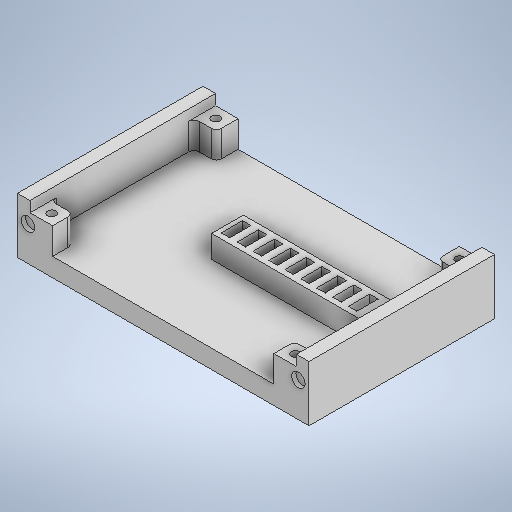
# Autodesk Inventor part: DisplayModuleHousing
Saved by Autodesk Inventor 2025.1 (Build 291241020, 241B)
## iProperties
Created: 2024-09-25
Part Number: DisplayModuleHousing
Material: Generic
Document SubType Name: Modeling
Designer: Si Teng Wu
Density: 1 g/cm^3
Appearance: Default
Author: Si Teng Wu
Autodesk Inventor part; units mm, degrees
ref_plane "YZ Plane" through (0, 0, 0) normal (1, 0, 0) x (0, 1, 0)
ref_plane "XZ Plane" through (0, 0, 0) normal (0, 1, 0) x (-1, 0, 0)
ref_plane "XY Plane" through (0, 0, 0) normal (0, 0, 1) x (1, 0, 0)
sketch "Sketch1" plane through (0, 0, 0) normal (0, 1, 0) x (-1, 0, 0)
  line L0 (55, 35) -> (-55, 35)
  line L1 (-55, 35) -> (-55, -35)
  line L2 (-55, -35) -> (55, -35)
  line L3 (55, -35) -> (55, 35)
  point P0 (0, 0)
  point P1 (-55, 0)
  point P2 (55, 0)
  dimension "d0" = 70
  dimension "d66" = 35
  dimension "d67" = 55
  dimension "d68" = 55
  constraints: 8 end point, 2 midpoint, 2 parallel, 1 horizontal, 1 perpendicular
  measures "d0" distance between parallel lines of L2 L0
  measures "d66" distance from line of L2 point (0, 0)
  measures "d67" distance of point (-55, 0) point (0, 0)
  measures "d68" distance of point (55, 0) point (0, 0)
extrude "Extrusion1" add sketch "Sketch1" along normal blind 21
sketch "Sketch2" plane through (0, 21, 0) normal (0, 1, 0) x (1, 0, 0)
  line L0 (-55, -35) -> (55, -35) projected
  line L1 (55, 35) -> (-55, 35) projected
  line L2 (50.25, -35) -> (-50.25, -35)
  line L3 (-50.25, -35) -> (-50.25, 35)
  line L4 (-50.25, 35) -> (50.25, 35)
  line L5 (50.25, 35) -> (50.25, -35)
  line L6 (-55, 35) -> (-55, -35) projected
  line L7 (55, -35) -> (55, 35) projected
  point P0 (0, 0)
  point P1 (-50.25, -35)
  dimension "d4" = 100.5
  dimension "d6" = 70
  dimension "d122" = 50.25
  constraints: 8 end point, 2 parallel, 2 point on line, 1 horizontal, 1 perpendicular
  measures "d4" distance between parallel lines of L3 L5
  measures "d6" distance between parallel lines of L1 L0
  measures "d122" distance from line of L3 point (0, 0)
extrude "Extrusion2" cut sketch "Sketch2" against normal blind 14 contours L3 L1 L5 L0
sketch "Sketch11" plane through (0, 7, 0) normal (0, 1, 0) x (1, 0, 0)
  line L0 (50.25, 35) -> (41.75, 35)
  line L1 (41.75, 35) -> (41.75, 26.8)
  line L2 (41.75, 26.8) -> (50.25, 26.8)
  line L3 (50.25, 26.8) -> (50.25, 35)
  circle A0 centre (46, 30.9) radius 1.6
  line L4 (50.25, 35) -> (50.25, -35) projected
  line L5 (50.25, -35) -> (41.75, -35)
  line L6 (41.75, -35) -> (41.75, -27.2)
  line L7 (41.75, -27.2) -> (50.25, -27.2)
  line L8 (50.25, -27.2) -> (50.25, -35)
  circle A1 centre (46, -31.1) radius 1.6
  line L9 (-41.75, 35) -> (-50.25, 35)
  line L10 (-50.25, 35) -> (-50.25, 26.8)
  line L11 (-50.25, 26.8) -> (-41.75, 26.8)
  line L12 (-41.75, 26.8) -> (-41.75, 35)
  circle A2 centre (-46, 30.8) radius 1.6
  line L13 (-50.25, 35) -> (50.25, 35) projected
  line L14 (-50.25, -35) -> (-50.25, 35) projected
  line L15 (-41.75, -35) -> (-50.25, -35)
  line L16 (-50.25, -35) -> (-50.25, -27.2)
  line L17 (-50.25, -27.2) -> (-41.75, -27.2)
  line L18 (-41.75, -27.2) -> (-41.75, -35)
  circle A3 centre (-46, -31.1) radius 1.6
  line L19 (50.25, -35) -> (-50.25, -35) projected
  point P0 (0, 0)
  point P1 (50.25, 30.9)
  point P2 (50.25, -8)
  point P3 (46, -35)
  point P4 (-41.75, 30.9)
  point P5 (-46, -35)
  point P6 (-50.25, -31.1)
  point P7 (50.25, -6)
  dimension "d74" = 8.5
  dimension "d75" = 8.2
  dimension "d76" = 3.2
  dimension "d77" = 4.1
  dimension "d78" = 4.25
  dimension "d79" = 8.5
  dimension "d80" = 7.8
  dimension "d81" = 4.25
  dimension "d82" = 3.9
  dimension "d83" = 3.2
  dimension "d84" = 8.5
  dimension "d85" = 8.2
  dimension "d86" = 3.2
  dimension "d87" = 4.2
  dimension "d89" = 7.8
  dimension "d90" = 3.9
  dimension "d91" = 3.2
  dimension "d92" = 4.25
  dimension "d93" = 8.5
  dimension "d115" = 4.25
  constraints: 32 end point, 8 parallel, 5 midpoint, 4 centre point, 4 horizontal, 4 perpendicular, 3 collinear, 1 point on line
  measures "d74" distance between parallel lines of L1 L3
  measures "d75" distance between parallel lines of L2 L0
  measures "d76" diameter of A0
  measures "d77" distance from line of L0 A0.centre
  measures "d78" distance of point (50.25, 30.9) A0.centre
  measures "d79" distance between parallel lines of L6 L4
  measures "d80" distance between parallel lines of L7 L5
  measures "d81" distance from line of L4 A1.centre
  measures "d82" distance of point (46, -35) A1.centre
  measures "d83" diameter of A1
  measures "d84" distance between parallel lines of L10 L12
  measures "d85" distance between parallel lines of L11 L9
  measures "d86" diameter of A2
  measures "d87" distance from line of L9 A2.centre
  measures "d89" distance between parallel lines of L17 L15
  measures "d90" distance of point (-46, -35) A3.centre
  measures "d91" diameter of A3
  measures "d92" distance from line of L16 A3.centre
  measures "d93" distance between parallel lines of L16 L18
  measures "d115" horizontal distance of point (-41.75, 30.9) A2.centre
extrude "Extrusion10" add sketch "Sketch11" along normal blind 10 contours L3 L2 L1 L0 | L12 L11 L10 L9 | L4 L5 L6 L7 | L17 L18 L15 L14
fillet "Fillet5" radius 2 8 edges at (41.75, 12, 27.2) (50.25, 12, 27.2) (41.75, 12, -26.8) (50.25, 12, -26.8) (-41.75, 12, -26.8) (-50.25, 12, -26.8) (-50.25, 12, 27.2) (-41.75, 12, 27.2)
sketch "Sketch12" plane through (-41.75, 7, 35) normal (0, 0, 1) x (1, 0, 0)
  circle A0 centre (-9.25, 6) radius 2.55
  line L0 (-8.5, 10) -> (0, 10) projected
  line L1 (-13.25, -7) -> (-13.25, 14) projected
  circle A1 centre (92.75, 6) radius 2.55
  line L2 (96.75, -7) -> (96.75, 14) projected
  line L3 (83.5, 10) -> (92, 10) projected
  point P0 (41.75, -7)
  dimension "d98" = 5.1
  dimension "d100" = 4
  dimension "d103" = 4
  dimension "d104" = 5.1
  dimension "d105" = 4
  dimension "d106" = 4
  constraints: 2 centre point
  measures "d98" diameter of A0
  measures "d100" distance from line of L0 A0.centre
  measures "d103" distance from line of L1 A0.centre
  measures "d104" diameter of A1
  measures "d105" distance from line of L2 A1.centre
  measures "d106" distance from line of L3 A1.centre
extrude "Extrusion11" cut sketch "Sketch12" against normal blind 1.6
sketch "Sketch13" plane through (55, 0, -35) normal (0, 0, -1) x (-1, 0, 0)
  circle A0 centre (106, 13) radius 2.55
  circle A1 centre (4, 13) radius 2.55
  line L0 (96.75, 17) -> (105.25, 17) projected
  line L1 (110, 0) -> (110, 21) projected
  line L2 (4.75, 17) -> (13.25, 17) projected
  line L3 (0, 0) -> (0, 21) projected
  point P0 (55, 0)
  dimension "d107" = 5.1
  dimension "d108" = 4
  dimension "d109" = 4
  dimension "d110" = 5.1
  dimension "d111" = 4
  dimension "d112" = 4
  constraints: 2 centre point
  measures "d107" diameter of A0
  measures "d108" distance from line of L0 A0.centre
  measures "d109" distance from line of L1 A0.centre
  measures "d110" diameter of A1
  measures "d111" distance from line of L2 A1.centre
  measures "d112" distance from line of L3 A1.centre
extrude "Extrusion12" cut sketch "Sketch13" against normal blind 1.6
sketch "Sketch14" plane through (-46, 7, 31.1) normal (0, 1, 0) x (1, 0, 0)
  point P0 (46, 31.1)
sketch "Sketch15" plane through (0, 7, 0) normal (0, 1, 0) x (1, 0, 0)
  circle A0 centre (46, -31.1) radius 1.6 projected
  circle A1 centre (46, -31.1) radius 1.6
  circle A2 centre (-46, -31.1) radius 1.6 projected
  circle A3 centre (-46, -31.1) radius 1.6
  circle A4 centre (-46, 30.8) radius 1.6 projected
  circle A5 centre (-46, 30.8) radius 1.6
  circle A6 centre (46, 30.9) radius 1.6 projected
  circle A7 centre (46, 30.9) radius 1.6
  point P0 (0, 0)
  constraints: 4 centre point, 4 coincident
extrude "Extrusion13" cut sketch "Sketch15" against normal through all
sketch "Sketch16" plane through (0, 0, 0) normal (0, -1, 0) x (1, 0, 0)
  line L0 (48.1, -27.6) -> (44.9, -27.6)
  line L1 (44.9, -27.6) -> (44.9, 27.6)
  line L2 (44.9, 27.6) -> (48.1, 27.6)
  line L3 (48.1, 27.6) -> (48.1, -27.6)
  line L4 (48.1, -27.6) -> (44.9, 27.6) construction
  line L5 (44.9, -27.6) -> (48.1, 27.6) construction
  line L6 (50.25, -24.8) -> (50.25, 25.2) projected
  line L7 (42.1, -27.6) -> (38.9, -27.6)
  line L8 (38.9, -27.6) -> (38.9, 27.6)
  line L9 (38.9, 27.6) -> (42.1, 27.6)
  line L10 (42.1, 27.6) -> (42.1, -27.6)
  line L11 (42.1, -27.6) -> (38.9, 27.6) construction
  line L12 (38.9, -27.6) -> (42.1, 27.6) construction
  line L13 (36.1, -27.6) -> (32.9, -27.6)
  line L14 (32.9, -27.6) -> (32.9, 27.6)
  line L15 (32.9, 27.6) -> (36.1, 27.6)
  line L16 (36.1, 27.6) -> (36.1, -27.6)
  line L17 (36.1, -27.6) -> (32.9, 27.6) construction
  line L18 (32.9, -27.6) -> (36.1, 27.6) construction
  line L19 (30.1, -27.6) -> (26.9, -27.6)
  line L20 (26.9, -27.6) -> (26.9, 27.6)
  line L21 (26.9, 27.6) -> (30.1, 27.6)
  line L22 (30.1, 27.6) -> (30.1, -27.6)
  line L23 (30.1, -27.6) -> (26.9, 27.6) construction
  line L24 (26.9, -27.6) -> (30.1, 27.6) construction
  line L25 (24.1, -27.6) -> (20.9, -27.6)
  line L26 (20.9, -27.6) -> (20.9, 27.6)
  line L27 (20.9, 27.6) -> (24.1, 27.6)
  line L28 (24.1, 27.6) -> (24.1, -27.6)
  line L29 (24.1, -27.6) -> (20.9, 27.6) construction
  line L30 (20.9, -27.6) -> (24.1, 27.6) construction
  line L31 (18.1, -27.6) -> (14.9, -27.6)
  line L32 (14.9, -27.6) -> (14.9, 27.6)
  line L33 (14.9, 27.6) -> (18.1, 27.6)
  line L34 (18.1, 27.6) -> (18.1, -27.6)
  line L35 (18.1, -27.6) -> (14.9, 27.6) construction
  line L36 (14.9, -27.6) -> (18.1, 27.6) construction
  line L37 (12.1, -27.6) -> (8.9, -27.6)
  line L38 (8.9, 27.6) -> (12.1, 27.6)
  line L39 (8.9, -27.6) -> (8.9, 27.6)
  line L40 (12.1, -27.6) -> (8.9, 27.6) construction
  line L41 (8.9, -27.6) -> (12.1, 27.6) construction
  line L42 (12.1, 27.6) -> (12.1, -27.6)
  line L43 (6.1, -27.6) -> (2.9, -27.6)
  line L44 (2.9, 27.6) -> (6.1, 27.6)
  line L45 (2.9, -27.6) -> (2.9, 27.6)
  line L46 (6.1, -27.6) -> (2.9, 27.6) construction
  line L47 (2.9, -27.6) -> (6.1, 27.6) construction
  line L48 (6.1, 27.6) -> (6.1, -27.6)
  line L49 (0.1, -27.6) -> (-3.1, -27.6)
  line L50 (-3.1, 27.6) -> (0.1, 27.6)
  line L51 (-3.1, -27.6) -> (-3.1, 27.6)
  line L52 (0.1, -27.6) -> (-3.1, 27.6) construction
  line L53 (-3.1, -27.6) -> (0.1, 27.6) construction
  line L54 (0.1, 27.6) -> (0.1, -27.6)
  line L55 (-5.9, -27.6) -> (-9.1, -27.6)
  line L56 (-9.1, 27.6) -> (-5.9, 27.6)
  line L57 (-9.1, -27.6) -> (-9.1, 27.6)
  line L58 (-5.9, -27.6) -> (-9.1, 27.6) construction
  line L59 (-9.1, -27.6) -> (-5.9, 27.6) construction
  line L60 (-5.9, 27.6) -> (-5.9, -27.6)
  line L61 (55, -35) -> (-55, -35) projected
  point P0 (46.5, 27.6)
  point P1 (40.5, 27.6)
  point P2 (34.5, 27.6)
  point P3 (28.5, 27.6)
  point P4 (22.5, 27.6)
  point P5 (16.5, 27.6)
  point P6 (10.5, 27.6)
  point P7 (4.5, 27.6)
  point P8 (-1.5, 27.6)
  point P9 (-7.5, 27.6)
  point P10 (46.5, -27.6)
  point P11 (40.5, 0)
  point P12 (46.5, 0)
  point P13 (34.5, 0)
  point P14 (40.5, 0)
  point P15 (28.5, 0)
  point P16 (34.5, 0)
  point P17 (22.5, 0)
  point P18 (28.5, 0)
  point P19 (16.5, 0)
  point P20 (22.5, 0)
  point P21 (10.5, 0)
  point P22 (16.5, 0)
  point P23 (4.5, 0)
  point P24 (10.5, 0)
  point P25 (-1.5, 0)
  point P26 (4.5, 0)
  point P27 (-7.5, 0)
  point P28 (-1.5, 0)
  point P29 (46.5, 0)
  dimension "d136" = 3.2
  dimension "d145" = 3.2
  dimension "d162" = 3.2
  dimension "d164" = 3.2
  dimension "d166" = 3.2
  dimension "d176" = 3.2
  dimension "d179" = 3.2
  dimension "d182" = 3.2
  dimension "d185" = 3.2
  dimension "d210" = 6
  dimension "d211" = 6
  dimension "d212" = 6
  dimension "d213" = 6
  dimension "d214" = 6
  dimension "d215" = 6
  dimension "d216" = 6
  dimension "d217" = 6
  dimension "d218" = 6
  dimension "d219" = 27.6
  dimension "d221" = 3.75
  dimension "d222" = 35
  constraints: 120 end point, 30 midpoint, 20 parallel, 19 collinear, 10 horizontal, 10 perpendicular
  measures "d136" distance between parallel lines of L1 L3
  measures "d145" distance between parallel lines of L14 L16
  measures "d162" distance between parallel lines of L20 L22
  measures "d164" distance between parallel lines of L26 L28
  measures "d166" distance between parallel lines of L32 L34
  measures "d176" distance between parallel lines of L39 L42
  measures "d179" distance between parallel lines of L45 L48
  measures "d182" distance between parallel lines of L51 L54
  measures "d185" distance between parallel lines of L57 L60
  measures "d210" distance of point (40.5, 0) point (46.5, 0)
  measures "d211" distance of point (34.5, 0) point (40.5, 0)
  measures "d212" distance of point (28.5, 0) point (34.5, 0)
  measures "d213" distance of point (22.5, 0) point (28.5, 0)
  measures "d214" distance of point (16.5, 0) point (22.5, 0)
  measures "d215" distance of point (10.5, 0) point (16.5, 0)
  measures "d216" distance of point (4.5, 0) point (10.5, 0)
  measures "d217" distance of point (-1.5, 0) point (4.5, 0)
  measures "d218" distance of point (-7.5, 0) point (-1.5, 0)
  measures "d219" distance from line of L0 point (46.5, 0)
  measures "d221" distance from line of L6 point (46.5, 0)
  measures "d222" distance from line of L61 point (46.5, 0)
extrude "Extrusion14" cut sketch "Sketch16" against normal blind 5
sketch "Sketch19" plane through (0, 7, 0) normal (0, 1, 0) x (1, 0, 0)
  line L0 (50.25, 35) -> (50.25, -35) projected
  line L1 (50.25, 6) -> (-10.75, 6)
  line L2 (-10.75, 6) -> (-10.75, -6)
  line L3 (-10.75, -6) -> (50.25, -6)
  line L4 (50.25, -6) -> (50.25, 6)
  line L5 (41.75, -35) -> (50.25, -35) projected
  point P0 (0, 0)
  dimension "d204" = 61
  dimension "d205" = 12
  dimension "d206" = 29
  constraints: 8 end point, 2 parallel, 1 horizontal, 1 perpendicular, 1 point on line
  measures "d204" distance between parallel lines of L2 L0
  measures "d205" distance between parallel lines of L3 L1
  measures "d206" distance between parallel lines of L5 L3
extrude "Extrusion16" add sketch "Sketch19" along normal blind 8.5
sketch "Sketch17" plane through (0, 0, 0) normal (0, -1, 0) x (1, 0, 0)
  line L0 (48.1, 27.6) -> (48.1, -27.6) projected
  line L1 (44.9, 4) -> (48.1, 4)
  line L2 (48.1, 4) -> (48.1, -4)
  line L3 (48.1, -4) -> (44.9, -4)
  line L4 (44.9, -4) -> (44.9, 4)
  line L5 (44.9, 4) -> (48.1, -4) construction
  line L6 (48.1, 4) -> (44.9, -4) construction
  line L7 (44.9, -27.6) -> (44.9, 27.6) projected
  line L8 (42.1, 27.6) -> (42.1, -27.6) projected
  line L9 (38.9, 4) -> (42.1, 4)
  line L10 (42.1, 4) -> (42.1, -4)
  line L11 (42.1, -4) -> (38.9, -4)
  line L12 (38.9, -4) -> (38.9, 4)
  line L13 (38.9, 4) -> (42.1, -4) construction
  line L14 (42.1, 4) -> (38.9, -4) construction
  line L15 (36.1, 27.6) -> (36.1, -27.6) projected
  line L16 (32.9, 4) -> (36.1, 4)
  line L17 (36.1, 4) -> (36.1, -4)
  line L18 (36.1, -4) -> (32.9, -4)
  line L19 (32.9, -4) -> (32.9, 4)
  line L20 (32.9, 4) -> (36.1, -4) construction
  line L21 (36.1, 4) -> (32.9, -4) construction
  line L22 (30.1, 27.6) -> (30.1, -27.6) projected
  line L23 (26.9, 4) -> (30.1, 4)
  line L24 (30.1, 4) -> (30.1, -4)
  line L25 (30.1, -4) -> (26.9, -4)
  line L26 (26.9, -4) -> (26.9, 4)
  line L27 (26.9, 4) -> (30.1, -4) construction
  line L28 (30.1, 4) -> (26.9, -4) construction
  line L29 (24.1, 27.6) -> (24.1, -27.6) projected
  line L30 (20.9, 4) -> (24.1, 4)
  line L31 (24.1, 4) -> (24.1, -4)
  line L32 (24.1, -4) -> (20.9, -4)
  line L33 (20.9, -4) -> (20.9, 4)
  line L34 (20.9, 4) -> (24.1, -4) construction
  line L35 (24.1, 4) -> (20.9, -4) construction
  line L36 (18.1, 27.6) -> (18.1, -27.6) projected
  line L37 (14.9, 4) -> (18.1, 4)
  line L38 (18.1, 4) -> (18.1, -4)
  line L39 (18.1, -4) -> (14.9, -4)
  line L40 (14.9, -4) -> (14.9, 4)
  line L41 (14.9, 4) -> (18.1, -4) construction
  line L42 (18.1, 4) -> (14.9, -4) construction
  line L43 (12.1, 27.6) -> (12.1, -27.6) projected
  line L44 (8.9, 4) -> (12.1, 4)
  line L45 (12.1, 4) -> (12.1, -4)
  line L46 (12.1, -4) -> (8.9, -4)
  line L47 (8.9, -4) -> (8.9, 4)
  line L48 (8.9, 4) -> (12.1, -4) construction
  line L49 (12.1, 4) -> (8.9, -4) construction
  line L50 (2.9, 4) -> (6.1, 4)
  line L51 (6.1, 4) -> (6.1, -4)
  line L52 (6.1, -4) -> (2.9, -4)
  line L53 (2.9, -4) -> (2.9, 4)
  line L54 (2.9, 4) -> (6.1, -4) construction
  line L55 (6.1, 4) -> (2.9, -4) construction
  line L56 (-3.1, 4) -> (0.1, 4)
  line L57 (0.1, 4) -> (0.1, -4)
  line L58 (0.1, -4) -> (-3.1, -4)
  line L59 (-3.1, -4) -> (-3.1, 4)
  line L60 (-3.1, 4) -> (0.1, -4) construction
  line L61 (0.1, 4) -> (-3.1, -4) construction
  line L62 (-5.9, 27.6) -> (-5.9, -27.6) projected
  line L63 (-9.1, 4) -> (-5.9, 4)
  line L64 (-5.9, 4) -> (-5.9, -4)
  line L65 (-5.9, -4) -> (-9.1, -4)
  line L66 (-9.1, -4) -> (-9.1, 4)
  line L67 (-9.1, 4) -> (-5.9, -4) construction
  line L68 (-5.9, 4) -> (-9.1, -4) construction
  line L69 (38.9, -27.6) -> (38.9, 27.6) projected
  line L70 (32.9, -27.6) -> (32.9, 27.6) projected
  line L71 (26.9, -27.6) -> (26.9, 27.6) projected
  line L72 (20.9, -27.6) -> (20.9, 27.6) projected
  line L73 (14.9, -27.6) -> (14.9, 27.6) projected
  line L74 (8.9, -27.6) -> (8.9, 27.6) projected
  line L75 (2.9, -27.6) -> (2.9, 27.6) projected
  line L76 (-3.1, -27.6) -> (-3.1, 27.6) projected
  line L77 (0.1, 27.6) -> (0.1, -27.6) projected
  line L78 (6.1, 27.6) -> (6.1, -27.6) projected
  line L79 (12.1, 27.6) -> (12.1, -27.6) projected
  line L80 (-9.1, -27.6) -> (-9.1, 27.6) projected
  line L81 (55, -35) -> (-55, -35) projected
  point P0 (0, 0)
  point P1 (46.5, 0)
  point P2 (40.5, 0)
  point P3 (34.5, 0)
  point P4 (28.5, 0)
  point P5 (22.5, 0)
  point P6 (16.5, 0)
  point P7 (10.5, 0)
  point P8 (4.5, 0)
  point P9 (-1.5, 0)
  point P10 (-7.5, 0)
  point P11 (46.5, -4)
  point P12 (42.1, 4)
  point P13 (48.1, 4)
  dimension "d200" = 4
  dimension "d201" = 35
  constraints: 120 end point, 23 collinear, 21 midpoint, 20 parallel, 16 point on line, 10 horizontal, 10 perpendicular
  measures "d200" distance of point (46.5, 0) point (46.5, -4)
  measures "d201" distance from line of L81 point (46.5, 0)
extrude "Extrusion15" cut sketch "Sketch17" against normal through all
sketch "Sketch18" plane through (50.25, 21, -35) normal (-1, 0, 0) x (0, 0, 1)
  point P0 (35, -21)
body "Solid1"
